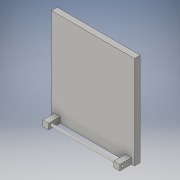
# Autodesk Inventor part: HingPartUno
Saved by Autodesk Inventor 2016 (Build 200138000, 138)
## iProperties
Created: 2017-02-17
Part Number: HingPartUno
Material: Generic
Document SubType Name: Modeling
Designer: RoboticsUser
Density: 1 g/cm^3
Appearance: Default
Author: RoboticsUser
Autodesk Inventor part; units mm, degrees
ref_plane "YZ Plane" through (0, 0, 0) normal (1, 0, 0) x (0, 1, 0)
ref_plane "XZ Plane" through (0, 0, 0) normal (0, 1, 0) x (-1, 0, 0)
ref_plane "XY Plane" through (0, 0, 0) normal (0, 0, 1) x (1, 0, 0)
sketch "Sketch1" plane through (0, 0, 0) normal (0, 0, 1) x (1, 0, 0)
  line L0 (0, 0) -> (45.212, 0)
  line L1 (45.212, 0) -> (45.212, 50.8)
  line L2 (45.212, 50.8) -> (0, 50.8)
  line L3 (0, 50.8) -> (0, 0)
  dimension "d0" = 45.212
  dimension "d1" = 50.8
  constraints: 8 end point, 2 parallel, 1 horizontal, 1 perpendicular
  measures "d0" distance of L2.end L1.end
  measures "d1" distance of L1.end L0.end
extrude "Extrusion1" add sketch "Sketch1" along normal blind 3.175
sketch "Sketch2" plane through (0, 0, 3.175) normal (0, 0, 1) x (1, 0, 0)
  line L0 (0, 0) -> (45.212, 0) projected
  line L1 (1.6002, 3.175) -> (4.7752, 3.175)
  line L2 (4.7752, 3.175) -> (4.7752, 0)
  line L3 (4.7752, 0) -> (1.6002, 0)
  line L4 (1.6002, 0) -> (1.6002, 3.175)
  dimension "d4" = 3.175
  dimension "d30" = 1.6002
  constraints: 8 end point, 2 parallel, 1 horizontal, 1 perpendicular, 1 point on line
  measures "d4" distance of L2.end L3.end
  measures "d30" distance of L0.start L3.end
extrude "Extrusion2" add sketch "Sketch2" along normal blind 6.35
sketch "Sketch3" plane through (0, 0, 3.175) normal (0, 0, 1) x (1, 0, 0)
  line L0 (4.7752, 0) -> (45.212, 0) projected
  line L1 (43.6118, 3.175) -> (40.4368, 3.175)
  line L2 (40.4368, 3.175) -> (40.4368, 0)
  line L3 (40.4368, 0) -> (43.6118, 0)
  line L4 (43.6118, 0) -> (43.6118, 3.175)
  line L5 (45.212, 0) -> (45.212, 50.8) projected
  point P0 (0, 0)
  dimension "d7" = 3.175
  dimension "d31" = 1.6002
  constraints: 8 end point, 2 parallel, 1 horizontal, 1 perpendicular, 1 point on line
  measures "d7" distance of L3.end L2.end
  measures "d31" distance between parallel lines of L5 L4
extrude "Extrusion3" add sketch "Sketch3" along normal blind 6.35
hole "Hole1" at (4.7752, 1.5748, 7.9248) direction (-1, 0, 0) diameter 1.27 end through all
hole "Hole2" at (40.4368, 1.5748, 7.9248) direction (1, 0, 0) diameter 1.27 end through all
sketch "Sketch4" plane through (4.7752, 0, 3.175) normal (1, 0, 0) x (0, 0, -1)
  point P0 (3.175, 0)
  point P1 (-4.7498, 1.5748)
extrude "Extrusion4" [suppressed]
sketch "Sketch5" plane through (4.7752, 0, 3.175) normal (1, 0, 0) x (0, 0, -1)
  point P0 (3.175, 0)
sketch "Sketch6" plane through (4.7752, 0, 3.175) normal (1, 0, 0) x (0, 0, -1)
  circle A0 centre (-4.7498, 1.5748) radius 0.635 projected
  circle A1 centre (-4.7498, 1.5748) radius 0.635
  point P0 (3.175, 0)
  constraints: 1 centre point, 1 coincident
extrude "Extrusion5" add sketch "Sketch6" along normal blind 35.6616
body "Solid1"
